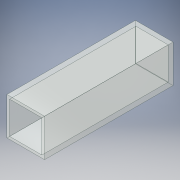
# Autodesk Inventor part: UG-752-30x30x120mm
Saved by Autodesk Inventor 2019 (Build 230136000, 136)
## iProperties
Created: 2016-07-06
Part Number: UG-752-30x30x120mm
Material: Glass
Document SubType Name: Modeling
Designer: voigt
Density: 2.18 g/cm^3
Appearance: Clear
Author: voigt
Autodesk Inventor part; units mm, degrees
ref_plane "YZ Plane" through (0, 0, 0) normal (1, 0, 0) x (0, 1, 0)
ref_plane "XZ Plane" through (0, 0, 0) normal (0, 1, 0) x (-1, 0, 0)
ref_plane "XY Plane" through (0, 0, 0) normal (0, 0, 1) x (1, 0, 0)
sketch "Sketch1" plane through (0, 0, 0) normal (0, 1, 0) x (-1, 0, 0)
  line L0 (0, -24.5) -> (0, 24.5) construction
  line L1 (-24.5, 0) -> (24.5, 0) construction
  line L2 (17.5, 17.5) -> (-17.5, 17.5)
  line L3 (-17.5, 17.5) -> (-17.5, -17.5)
  line L4 (-17.5, -17.5) -> (17.5, -17.5)
  line L5 (17.5, -17.5) -> (17.5, 17.5)
  line L6 (15, 15) -> (-15, 15)
  line L7 (-15, 15) -> (-15, -15)
  line L8 (-15, -15) -> (15, -15)
  line L9 (15, -15) -> (15, 15)
  point P0 (0, 0)
  dimension "d0" = 35
  dimension "d1" = 35
  dimension "d2" = 30
  dimension "d3" = 30
  constraints: 16 end point, 4 parallel, 2 horizontal, 2 perpendicular, 4 other
  measures "d0" distance of L3.end L4.end
  measures "d1" distance of L2.end L3.end
  measures "d2" distance of L8.end L7.end
  measures "d3" distance of L7.end L6.end
extrude "Extrusion1" add sketch "Sketch1" along normal blind 117.5
sketch "Sketch2" plane through (0, 117.5, 0) normal (0, 1, 0) x (1, 0, 0)
  line L0 (-17.5, 17.5) -> (-17.5, -17.5) projected
  line L1 (-17.5, -17.5) -> (17.5, -17.5) projected
  line L2 (17.5, -17.5) -> (17.5, 17.5) projected
  line L3 (17.5, 17.5) -> (-17.5, 17.5) projected
  point P0 (0, 0)
extrude "Extrusion2" add sketch "Sketch2" along normal blind 2
body "Solid1"
